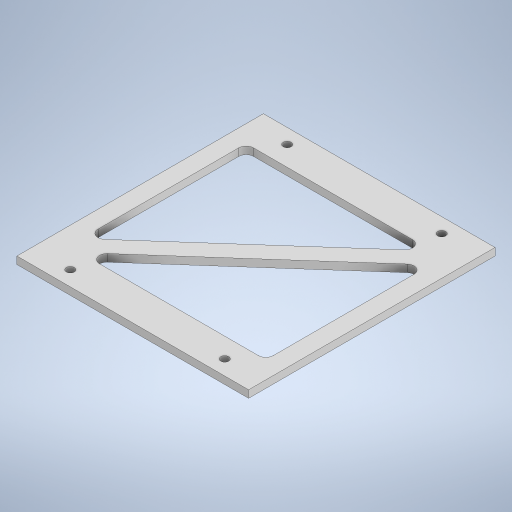
# Autodesk Inventor part: FrontPanel
Saved by Autodesk Inventor 2023 (Build 270158000, 158)
## iProperties
Created: 2022-07-23
Part Number: FrontPanel
Material: Generic
Document SubType Name: Modeling
Designer: Aditya Bansal
Density: 1 g/cm^3
Appearance: Default
Author: Aditya Bansal
Autodesk Inventor part; units mm, degrees
ref_plane "YZ Plane" through (0, 0, 0) normal (1, 0, 0) x (0, 1, 0)
ref_plane "XZ Plane" through (0, 0, 0) normal (0, 1, 0) x (-1, 0, 0)
ref_plane "XY Plane" through (0, 0, 0) normal (0, 0, 1) x (1, 0, 0)
sketch "Sketch1" plane through (0, 0, 0) normal (0, 1, 0) x (-1, 0, 0)
  line L0 (0, 0) -> (94, 0)
  line L1 (94, -100) -> (0, -100)
  line L2 (0, -100) -> (0, 0)
  line L3 (94, 0) -> (0, 0) construction
  line L4 (0, 0) -> (0, -9) construction
  line L5 (0, -9) -> (94, -9) construction
  line L6 (94, -9) -> (94, 0) construction
  line L7 (0, -100) -> (94, -100) construction
  line L8 (94, -100) -> (94, -91) construction
  line L9 (94, -91) -> (0, -91) construction
  line L10 (0, -91) -> (0, -100) construction
  line L11 (94, 0) -> (94, -100)
  circle A0 centre (78.3333, -6) radius 1.6
  circle A1 centre (15.6667, -6) radius 1.6
  circle A2 centre (78.3333, -94) radius 1.6
  circle A3 centre (15.6667, -94) radius 1.6
  line L12 (82.3582, -14) -> (7, -80.7604)
  line L13 (7, -80.7604) -> (7, -14)
  line L14 (7, -14) -> (82.3582, -14)
  line L15 (87, -19.2396) -> (11.6418, -86)
  line L16 (11.6418, -86) -> (87, -86)
  line L17 (87, -86) -> (87, -19.2396)
  line L18 (82.3582, -14) -> (87, -19.2396) construction
  line L19 (11.6418, -86) -> (7, -80.7604) construction
  dimension "d0" = 100
  dimension "d1" = 9
  dimension "d2" = 3
  dimension "d3" = 3.2
  dimension "d4" = 15.6667
  dimension "d5" = 62.6667
  dimension "d6" = 94
  dimension "d7" = 3
  dimension "d10" = 7
  dimension "d11" = 7
  dimension "d12" = 7
  dimension "d13" = 5
  dimension "d14" = 5
  constraints: 41 end point, 7 parallel, 7 perpendicular, 4 centre point, 3 equal radius, 3 horizontal, 2 collinear, 2 horizontal alignment, 2 vertical alignment, 1 point on line, 1 vertical
  measures "d0" distance of L0.end L1.start
  measures "d1" distance between parallel lines of L1 L9
  measures "d2" distance from line of L5 A0.centre
  measures "d3" diameter of A0
  measures "d4" distance from line of L6 A0.centre
  measures "d5" distance of A1.centre A0.centre
  measures "d6" distance of L1.start L1.end
  measures "d7" distance from line of L9 A2.centre
  measures "d10" distance between parallel lines of L15 L12
  measures "d11" distance between parallel lines of L11 L17
  measures "d12" distance between parallel lines of L2 L13
  measures "d13" distance between parallel lines of L5 L14
  measures "d14" distance between parallel lines of L9 L16
extrude "Extrusion1" add sketch "Sketch1" along normal blind 3
fillet "Fillet1" radius 3 6 edges at (-82.3582, 1.5, -14) (-7, 1.5, -14) (-7, 1.5, -80.7604) (-87, 1.5, -19.2396) (-11.6418, 1.5, -86) (-87, 1.5, -86)
equation "\"d4\" = 0.166667 * d6"
equation "\"d5\" = 4 * d4"
equation "\"d11\" = d10"
equation "\"d12\" = d11"
equation "\"d14\" = d13"
body "Solid1"
